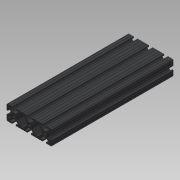
# Autodesk Inventor part: 1545
Saved by Autodesk Inventor 2013 (Build 170138000, 138)
## iProperties
Company: 80/20 Inc.
Created: 2014-04-23
Part Number: 1545
Material: Generic
Document SubType Name: Modeling
Density: 1 g/cm^3
Vendor: 80/20 Inc.
Engineer: Ross Bowman
Designer: Ross Bowman
Catalog Web Link: 8020.net
Material: 6105-T5 Aluminum
Author: Ross Bowman
Keywords: 80/20 , 8020 , T-Slot , Extrusion
Autodesk Inventor part; units mm, degrees
ref_plane "YZ Plane" through (0, 0, 0) normal (1, 0, 0) x (0, 1, 0)
ref_plane "XZ Plane" through (0, 0, 0) normal (0, 1, 0) x (-1, 0, 0)
ref_plane "XY Plane" through (0, 0, 0) normal (0, 0, 1) x (1, 0, 0)
sketch "Sketch1" plane through (0, 0, 0) normal (0, 0, 1) x (1, 0, 0)
  circle A0 centre (-38.1, 0) radius 3.3274
  arc A1 (-7.8382, -5.2928) -> (-6.447, -1.9341) centre (-11.1968, -1.9341) ccw
  line L0 (-16.8269, -14.2815) -> (-7.8382, -5.2928)
  arc A2 (-20.9826, -14.2815) -> (-16.8269, -14.2815) centre (-18.9048, -12.2036) ccw
  line L1 (-29.9713, -5.2928) -> (-20.9826, -14.2815)
  arc A3 (-31.3625, -1.9341) -> (-29.9713, -5.2928) centre (-26.6127, -1.9341) ccw
  line L2 (-31.3625, 1.9341) -> (-31.3625, -1.9341)
  arc A4 (-29.9713, 5.2928) -> (-31.3625, 1.9341) centre (-26.6127, 1.9341) ccw
  line L3 (-20.9826, 14.2815) -> (-29.9713, 5.2928)
  arc A5 (-16.8269, 14.2815) -> (-20.9826, 14.2815) centre (-18.9048, 12.2036) ccw
  line L4 (-7.8382, 5.2928) -> (-16.8269, 14.2815)
  arc A6 (-6.447, 1.9341) -> (-7.8382, 5.2928) centre (-11.1968, 1.9341) ccw
  line L5 (-6.447, -1.9341) -> (-6.447, 1.9341)
  arc A7 (6.447, -1.9341) -> (7.8382, -5.2928) centre (11.1968, -1.9341) ccw
  line L6 (6.447, 1.9341) -> (6.447, -1.9341)
  arc A8 (7.8382, 5.2928) -> (6.447, 1.9341) centre (11.1968, 1.9341) ccw
  line L7 (16.8269, 14.2815) -> (7.8382, 5.2928)
  arc A9 (20.9826, 14.2815) -> (16.8269, 14.2815) centre (18.9048, 12.2036) ccw
  line L8 (29.9713, 5.2928) -> (20.9826, 14.2815)
  arc A10 (31.3625, 1.9341) -> (29.9713, 5.2928) centre (26.6127, 1.9341) ccw
  line L9 (31.3625, -1.9341) -> (31.3625, 1.9341)
  arc A11 (29.9713, -5.2928) -> (31.3625, -1.9341) centre (26.6127, -1.9341) ccw
  line L10 (20.9826, -14.2815) -> (29.9713, -5.2928)
  arc A12 (16.8269, -14.2815) -> (20.9826, -14.2815) centre (18.9048, -12.2036) ccw
  line L11 (7.8382, -5.2928) -> (16.8269, -14.2815)
  circle A13 centre (0, 0) radius 3.3274
  circle A14 centre (38.1, 0) radius 3.3274
  arc A15 (9.1305, -14.986) -> (10.0195, -14.097) centre (9.1305, -14.097) ccw
  line L12 (9.1305, -14.986) -> (5.6388, -14.986)
  arc A16 (5.6388, -14.986) -> (4.064, -16.5608) centre (5.6388, -16.5608) ccw
  line L13 (4.064, -16.5608) -> (4.064, -17.4752)
  arc A17 (4.064, -17.4752) -> (5.6388, -19.05) centre (5.6388, -17.4752) ccw
  line L14 (5.6388, -19.05) -> (8.0238, -19.05)
  arc A18 (9.5478, -19.05) -> (8.0238, -19.05) centre (8.7858, -19.05) ccw
  line L15 (9.5478, -19.05) -> (13.9845, -19.05)
  arc A19 (15.5085, -19.05) -> (13.9845, -19.05) centre (14.7465, -19.05) ccw
  line L16 (15.5085, -19.05) -> (22.301, -19.05)
  arc A20 (23.825, -19.05) -> (22.301, -19.05) centre (23.063, -19.05) ccw
  line L17 (23.825, -19.05) -> (28.6534, -19.05)
  arc A21 (30.1774, -19.05) -> (28.6534, -19.05) centre (29.4154, -19.05) ccw
  line L18 (30.1774, -19.05) -> (32.4612, -19.05)
  arc A22 (32.4612, -19.05) -> (34.036, -17.4752) centre (32.4612, -17.4752) ccw
  line L19 (34.036, -17.4752) -> (34.036, -16.5608)
  arc A23 (34.036, -16.5608) -> (32.4612, -14.986) centre (32.4612, -16.5608) ccw
  line L20 (32.4612, -14.986) -> (28.7209, -14.986)
  arc A24 (27.8319, -14.097) -> (28.7209, -14.986) centre (28.7209, -14.097) ccw
  line L21 (27.8319, -14.097) -> (27.8319, -13.5478)
  arc A25 (28.0922, -12.9192) -> (27.8319, -13.5478) centre (28.7209, -13.5478) ccw
  line L22 (28.0922, -12.9192) -> (32.8638, -8.1476)
  arc A26 (36.2224, -6.7564) -> (32.8638, -8.1476) centre (36.2224, -11.5062) ccw
  line L23 (36.2224, -6.7564) -> (40.2439, -6.7564)
  arc A27 (43.6025, -8.3762) -> (40.2439, -6.7564) centre (40.0255, -11.5012) ccw
  line L24 (43.6025, -8.3762) -> (48.1455, -12.9192)
  arc A28 (48.4059, -13.5478) -> (48.1455, -12.9192) centre (47.5169, -13.5478) ccw
  line L25 (48.4059, -13.5478) -> (48.4059, -14.097)
  arc A29 (47.5169, -14.986) -> (48.4059, -14.097) centre (47.5169, -14.097) ccw
  line L26 (47.5169, -14.986) -> (43.7388, -14.986)
  arc A30 (43.7388, -14.986) -> (42.164, -16.5608) centre (43.7388, -16.5608) ccw
  line L27 (42.164, -16.5608) -> (42.164, -17.4752)
  arc A31 (42.164, -17.4752) -> (43.7388, -19.05) centre (43.7388, -17.4752) ccw
  line L28 (43.7388, -19.05) -> (46.1257, -19.05)
  arc A32 (47.6497, -19.05) -> (46.1257, -19.05) centre (46.8877, -19.05) ccw
  line L29 (47.6497, -19.05) -> (52.4761, -19.05)
  arc A33 (53.9265, -19.0499) -> (52.4761, -19.05) centre (53.2013, -19.0141) ccw
  arc A34 (53.9265, -19.0499) -> (57.1499, -15.8265) centre (53.9046, -15.8046) ccw
  arc A35 (57.15, -14.3761) -> (57.1499, -15.8265) centre (57.1141, -15.1013) ccw
  line L30 (57.15, -14.3761) -> (57.15, -9.5497)
  arc A36 (57.15, -8.0257) -> (57.15, -9.5497) centre (57.15, -8.7877) ccw
  line L31 (57.15, -8.0257) -> (57.15, -5.6388)
  arc A37 (57.15, -5.6388) -> (55.5752, -4.064) centre (55.5752, -5.6388) ccw
  line L32 (55.5752, -4.064) -> (54.6608, -4.064)
  arc A38 (54.6608, -4.064) -> (53.086, -5.6388) centre (54.6608, -5.6388) ccw
  line L33 (53.086, -5.6388) -> (53.086, -9.4169)
  arc A39 (52.2159, -10.287) -> (53.086, -9.4169) centre (52.2159, -9.4169) ccw
  line L34 (52.2159, -10.287) -> (51.6289, -10.287)
  arc A40 (51.0003, -10.0266) -> (51.6289, -10.287) centre (51.6289, -9.398) ccw
  line L35 (51.0003, -10.0266) -> (46.2476, -5.2739)
  arc A41 (44.8564, -1.9153) -> (46.2476, -5.2739) centre (49.6062, -1.9153) ccw
  line L36 (44.8564, -1.9153) -> (44.8564, 1.9153)
  arc A42 (46.2476, 5.2739) -> (44.8564, 1.9153) centre (49.6062, 1.9153) ccw
  line L37 (46.2476, 5.2739) -> (51.0003, 10.0266)
  arc A43 (51.6289, 10.287) -> (51.0003, 10.0266) centre (51.6289, 9.398) ccw
  line L38 (51.6289, 10.287) -> (52.2159, 10.287)
  arc A44 (53.086, 9.4169) -> (52.2159, 10.287) centre (52.2159, 9.4169) ccw
  line L39 (53.086, 9.4169) -> (53.086, 5.6388)
  arc A45 (53.086, 5.6388) -> (54.6608, 4.064) centre (54.6608, 5.6388) ccw
  line L40 (54.6608, 4.064) -> (55.5752, 4.064)
  arc A46 (55.5752, 4.064) -> (57.15, 5.6388) centre (55.5752, 5.6388) ccw
  line L41 (57.15, 5.6388) -> (57.15, 8.0257)
  arc A47 (57.15, 9.5497) -> (57.15, 8.0257) centre (57.15, 8.7877) ccw
  line L42 (57.15, 9.5497) -> (57.15, 14.3761)
  arc A48 (57.1499, 15.8265) -> (57.15, 14.3761) centre (57.1141, 15.1013) ccw
  arc A49 (57.1499, 15.8265) -> (53.9265, 19.0499) centre (53.9046, 15.8046) ccw
  arc A50 (52.4761, 19.05) -> (53.9265, 19.0499) centre (53.2013, 19.0141) ccw
  line L43 (52.4761, 19.05) -> (47.6497, 19.05)
  arc A51 (46.1257, 19.05) -> (47.6497, 19.05) centre (46.8877, 19.05) ccw
  line L44 (46.1257, 19.05) -> (43.7388, 19.05)
  arc A52 (43.7388, 19.05) -> (42.164, 17.4752) centre (43.7388, 17.4752) ccw
  line L45 (42.164, 17.4752) -> (42.164, 16.5608)
  arc A53 (42.164, 16.5608) -> (43.7388, 14.986) centre (43.7388, 16.5608) ccw
  line L46 (43.7388, 14.986) -> (47.5169, 14.986)
  arc A54 (48.4059, 14.097) -> (47.5169, 14.986) centre (47.5169, 14.097) ccw
  line L47 (48.4059, 14.097) -> (48.4059, 13.5478)
  arc A55 (48.1455, 12.9192) -> (48.4059, 13.5478) centre (47.5169, 13.5478) ccw
  line L48 (48.1455, 12.9192) -> (43.6025, 8.3762)
  arc A56 (40.2439, 6.7564) -> (43.6025, 8.3762) centre (40.0255, 11.5012) ccw
  line L49 (40.2439, 6.7564) -> (36.2224, 6.7564)
  arc A57 (32.8638, 8.1476) -> (36.2224, 6.7564) centre (36.2224, 11.5062) ccw
  line L50 (32.8638, 8.1476) -> (28.0922, 12.9192)
  arc A58 (27.8319, 13.5478) -> (28.0922, 12.9192) centre (28.7209, 13.5478) ccw
  line L51 (27.8319, 13.5478) -> (27.8319, 14.097)
  arc A59 (28.7209, 14.986) -> (27.8319, 14.097) centre (28.7209, 14.097) ccw
  line L52 (28.7209, 14.986) -> (32.4612, 14.986)
  arc A60 (32.4612, 14.986) -> (34.036, 16.5608) centre (32.4612, 16.5608) ccw
  line L53 (34.036, 16.5608) -> (34.036, 17.4752)
  arc A61 (34.036, 17.4752) -> (32.4612, 19.05) centre (32.4612, 17.4752) ccw
  line L54 (32.4612, 19.05) -> (30.1774, 19.05)
  arc A62 (28.6534, 19.05) -> (30.1774, 19.05) centre (29.4154, 19.05) ccw
  line L55 (28.6534, 19.05) -> (23.825, 19.05)
  arc A63 (22.301, 19.05) -> (23.825, 19.05) centre (23.063, 19.05) ccw
  line L56 (22.301, 19.05) -> (15.5085, 19.05)
  arc A64 (13.9845, 19.05) -> (15.5085, 19.05) centre (14.7465, 19.05) ccw
  line L57 (13.9845, 19.05) -> (9.5478, 19.05)
  arc A65 (8.0238, 19.05) -> (9.5478, 19.05) centre (8.7858, 19.05) ccw
  line L58 (8.0238, 19.05) -> (5.6388, 19.05)
  arc A66 (5.6388, 19.05) -> (4.064, 17.4752) centre (5.6388, 17.4752) ccw
  line L59 (4.064, 17.4752) -> (4.064, 16.5608)
  arc A67 (4.064, 16.5608) -> (5.6388, 14.986) centre (5.6388, 16.5608) ccw
  line L60 (5.6388, 14.986) -> (9.1305, 14.986)
  arc A68 (10.0195, 14.097) -> (9.1305, 14.986) centre (9.1305, 14.097) ccw
  line L61 (10.0195, 14.097) -> (10.0195, 13.5896)
  arc A69 (9.7591, 12.961) -> (10.0195, 13.5896) centre (9.1305, 13.5896) ccw
  line L62 (9.7591, 12.961) -> (4.9457, 8.1476)
  arc A70 (1.5871, 6.7564) -> (4.9457, 8.1476) centre (1.5871, 11.5062) ccw
  line L63 (1.5871, 6.7564) -> (-1.5871, 6.7564)
  arc A71 (-4.9457, 8.1476) -> (-1.5871, 6.7564) centre (-1.5871, 11.5062) ccw
  line L64 (-4.9457, 8.1476) -> (-9.7591, 12.961)
  arc A72 (-10.0195, 13.5896) -> (-9.7591, 12.961) centre (-9.1305, 13.5896) ccw
  line L65 (-10.0195, 13.5896) -> (-10.0195, 14.097)
  arc A73 (-9.1305, 14.986) -> (-10.0195, 14.097) centre (-9.1305, 14.097) ccw
  line L66 (-9.1305, 14.986) -> (-5.6388, 14.986)
  arc A74 (-5.6388, 14.986) -> (-4.064, 16.5608) centre (-5.6388, 16.5608) ccw
  line L67 (-4.064, 16.5608) -> (-4.064, 17.4752)
  arc A75 (-4.064, 17.4752) -> (-5.6388, 19.05) centre (-5.6388, 17.4752) ccw
  line L68 (-5.6388, 19.05) -> (-8.0238, 19.05)
  arc A76 (-9.5478, 19.05) -> (-8.0238, 19.05) centre (-8.7858, 19.05) ccw
  line L69 (-9.5478, 19.05) -> (-13.9845, 19.05)
  arc A77 (-15.5085, 19.05) -> (-13.9845, 19.05) centre (-14.7465, 19.05) ccw
  line L70 (-15.5085, 19.05) -> (-22.301, 19.05)
  arc A78 (-23.825, 19.05) -> (-22.301, 19.05) centre (-23.063, 19.05) ccw
  line L71 (-23.825, 19.05) -> (-28.6534, 19.05)
  arc A79 (-30.1774, 19.05) -> (-28.6534, 19.05) centre (-29.4154, 19.05) ccw
  line L72 (-30.1774, 19.05) -> (-32.4612, 19.05)
  arc A80 (-32.4612, 19.05) -> (-34.036, 17.4752) centre (-32.4612, 17.4752) ccw
  line L73 (-34.036, 17.4752) -> (-34.036, 16.5608)
  arc A81 (-34.036, 16.5608) -> (-32.4612, 14.986) centre (-32.4612, 16.5608) ccw
  line L74 (-32.4612, 14.986) -> (-28.7209, 14.986)
  arc A82 (-27.8319, 14.097) -> (-28.7209, 14.986) centre (-28.7209, 14.097) ccw
  line L75 (-27.8319, 14.097) -> (-27.8319, 13.5478)
  arc A83 (-28.0922, 12.9192) -> (-27.8319, 13.5478) centre (-28.7209, 13.5478) ccw
  line L76 (-28.0922, 12.9192) -> (-32.8638, 8.1476)
  arc A84 (-36.2224, 6.7564) -> (-32.8638, 8.1476) centre (-36.2224, 11.5062) ccw
  line L77 (-36.2224, 6.7564) -> (-40.2439, 6.7564)
  arc A85 (-43.6025, 8.3762) -> (-40.2439, 6.7564) centre (-40.0255, 11.5012) ccw
  line L78 (-43.6025, 8.3762) -> (-48.1455, 12.9192)
  arc A86 (-48.4059, 13.5478) -> (-48.1455, 12.9192) centre (-47.5169, 13.5478) ccw
  line L79 (-48.4059, 13.5478) -> (-48.4059, 14.097)
  arc A87 (-47.5169, 14.986) -> (-48.4059, 14.097) centre (-47.5169, 14.097) ccw
  line L80 (-47.5169, 14.986) -> (-43.7388, 14.986)
  arc A88 (-43.7388, 14.986) -> (-42.164, 16.5608) centre (-43.7388, 16.5608) ccw
  line L81 (-42.164, 16.5608) -> (-42.164, 17.4752)
  arc A89 (-42.164, 17.4752) -> (-43.7388, 19.05) centre (-43.7388, 17.4752) ccw
  line L82 (-43.7388, 19.05) -> (-46.1257, 19.05)
  arc A90 (-47.6497, 19.05) -> (-46.1257, 19.05) centre (-46.8877, 19.05) ccw
  line L83 (-47.6497, 19.05) -> (-52.4761, 19.05)
  arc A91 (-53.9265, 19.0499) -> (-52.4761, 19.05) centre (-53.2013, 19.0141) ccw
  arc A92 (-53.9265, 19.0499) -> (-57.1499, 15.8265) centre (-53.9046, 15.8046) ccw
  arc A93 (-57.15, 14.3761) -> (-57.1499, 15.8265) centre (-57.1141, 15.1013) ccw
  line L84 (-57.15, 14.3761) -> (-57.15, 9.5497)
  arc A94 (-57.15, 8.0257) -> (-57.15, 9.5497) centre (-57.15, 8.7877) ccw
  line L85 (-57.15, 8.0257) -> (-57.15, 5.6388)
  arc A95 (-57.15, 5.6388) -> (-55.5752, 4.064) centre (-55.5752, 5.6388) ccw
  line L86 (-55.5752, 4.064) -> (-54.6608, 4.064)
  arc A96 (-54.6608, 4.064) -> (-53.086, 5.6388) centre (-54.6608, 5.6388) ccw
  line L87 (-53.086, 5.6388) -> (-53.086, 9.4169)
  arc A97 (-52.2159, 10.287) -> (-53.086, 9.4169) centre (-52.2159, 9.4169) ccw
  line L88 (-52.2159, 10.287) -> (-51.6289, 10.287)
  arc A98 (-51.0003, 10.0266) -> (-51.6289, 10.287) centre (-51.6289, 9.398) ccw
  line L89 (-51.0003, 10.0266) -> (-46.2476, 5.2739)
  arc A99 (-44.8564, 1.9153) -> (-46.2476, 5.2739) centre (-49.6062, 1.9153) ccw
  line L90 (-44.8564, 1.9153) -> (-44.8564, -1.9153)
  arc A100 (-46.2476, -5.2739) -> (-44.8564, -1.9153) centre (-49.6062, -1.9153) ccw
  line L91 (-46.2476, -5.2739) -> (-51.0003, -10.0266)
  arc A101 (-51.6289, -10.287) -> (-51.0003, -10.0266) centre (-51.6289, -9.398) ccw
  line L92 (-51.6289, -10.287) -> (-52.2159, -10.287)
  arc A102 (-53.086, -9.4169) -> (-52.2159, -10.287) centre (-52.2159, -9.4169) ccw
  line L93 (-53.086, -9.4169) -> (-53.086, -5.6388)
  arc A103 (-53.086, -5.6388) -> (-54.6608, -4.064) centre (-54.6608, -5.6388) ccw
  line L94 (-54.6608, -4.064) -> (-55.5752, -4.064)
  arc A104 (-55.5752, -4.064) -> (-57.15, -5.6388) centre (-55.5752, -5.6388) ccw
  line L95 (-57.15, -5.6388) -> (-57.15, -8.0257)
  arc A105 (-57.15, -9.5497) -> (-57.15, -8.0257) centre (-57.15, -8.7877) ccw
  line L96 (-57.15, -9.5497) -> (-57.15, -14.3761)
  arc A106 (-57.1499, -15.8265) -> (-57.15, -14.3761) centre (-57.1141, -15.1013) ccw
  arc A107 (-57.1499, -15.8265) -> (-53.9265, -19.0499) centre (-53.9046, -15.8046) ccw
  arc A108 (-52.4761, -19.05) -> (-53.9265, -19.0499) centre (-53.2013, -19.0141) ccw
  line L97 (-52.4761, -19.05) -> (-47.6497, -19.05)
  arc A109 (-46.1257, -19.05) -> (-47.6497, -19.05) centre (-46.8877, -19.05) ccw
  line L98 (-46.1257, -19.05) -> (-43.7388, -19.05)
  arc A110 (-43.7388, -19.05) -> (-42.164, -17.4752) centre (-43.7388, -17.4752) ccw
  line L99 (-42.164, -17.4752) -> (-42.164, -16.5608)
  arc A111 (-42.164, -16.5608) -> (-43.7388, -14.986) centre (-43.7388, -16.5608) ccw
  line L100 (-43.7388, -14.986) -> (-47.5169, -14.986)
  arc A112 (-48.4059, -14.097) -> (-47.5169, -14.986) centre (-47.5169, -14.097) ccw
  line L101 (-48.4059, -14.097) -> (-48.4059, -13.5478)
  arc A113 (-48.1455, -12.9192) -> (-48.4059, -13.5478) centre (-47.5169, -13.5478) ccw
  line L102 (-48.1455, -12.9192) -> (-43.6025, -8.3762)
  arc A114 (-40.2439, -6.7564) -> (-43.6025, -8.3762) centre (-40.0255, -11.5012) ccw
  line L103 (-40.2439, -6.7564) -> (-36.2224, -6.7564)
  arc A115 (-32.8638, -8.1476) -> (-36.2224, -6.7564) centre (-36.2224, -11.5062) ccw
  line L104 (-32.8638, -8.1476) -> (-28.0922, -12.9192)
  arc A116 (-27.8319, -13.5478) -> (-28.0922, -12.9192) centre (-28.7209, -13.5478) ccw
  line L105 (-27.8319, -13.5478) -> (-27.8319, -14.097)
  arc A117 (-28.7209, -14.986) -> (-27.8319, -14.097) centre (-28.7209, -14.097) ccw
  line L106 (-28.7209, -14.986) -> (-32.4612, -14.986)
  arc A118 (-32.4612, -14.986) -> (-34.036, -16.5608) centre (-32.4612, -16.5608) ccw
  line L107 (-34.036, -16.5608) -> (-34.036, -17.4752)
  arc A119 (-34.036, -17.4752) -> (-32.4612, -19.05) centre (-32.4612, -17.4752) ccw
  line L108 (-32.4612, -19.05) -> (-30.1774, -19.05)
  arc A120 (-28.6534, -19.05) -> (-30.1774, -19.05) centre (-29.4154, -19.05) ccw
  line L109 (-28.6534, -19.05) -> (-23.825, -19.05)
  arc A121 (-22.301, -19.05) -> (-23.825, -19.05) centre (-23.063, -19.05) ccw
  line L110 (-22.301, -19.05) -> (-15.5085, -19.05)
  arc A122 (-13.9845, -19.05) -> (-15.5085, -19.05) centre (-14.7465, -19.05) ccw
  line L111 (-13.9845, -19.05) -> (-9.5478, -19.05)
  arc A123 (-8.0238, -19.05) -> (-9.5478, -19.05) centre (-8.7858, -19.05) ccw
  line L112 (-8.0238, -19.05) -> (-5.6388, -19.05)
  arc A124 (-5.6388, -19.05) -> (-4.064, -17.4752) centre (-5.6388, -17.4752) ccw
  line L113 (-4.064, -17.4752) -> (-4.064, -16.5608)
  arc A125 (-4.064, -16.5608) -> (-5.6388, -14.986) centre (-5.6388, -16.5608) ccw
  line L114 (-5.6388, -14.986) -> (-9.1305, -14.986)
  arc A126 (-10.0195, -14.097) -> (-9.1305, -14.986) centre (-9.1305, -14.097) ccw
  line L115 (-10.0195, -14.097) -> (-10.0195, -13.5896)
  arc A127 (-9.7591, -12.961) -> (-10.0195, -13.5896) centre (-9.1305, -13.5896) ccw
  line L116 (-9.7591, -12.961) -> (-4.9457, -8.1476)
  arc A128 (-1.5871, -6.7564) -> (-4.9457, -8.1476) centre (-1.5871, -11.5062) ccw
  line L117 (-1.5871, -6.7564) -> (1.5871, -6.7564)
  arc A129 (4.9457, -8.1476) -> (1.5871, -6.7564) centre (1.5871, -11.5062) ccw
  line L118 (4.9457, -8.1476) -> (9.7591, -12.961)
  arc A130 (10.0195, -13.5896) -> (9.7591, -12.961) centre (9.1305, -13.5896) ccw
  line L119 (10.0195, -13.5896) -> (10.0195, -14.097)
  constraints: 256 point on circle, 240 end point, 131 centre point
extrude "Extrusion1" add sketch "Sketch1" against normal blind 304.8
body "Solid1"
